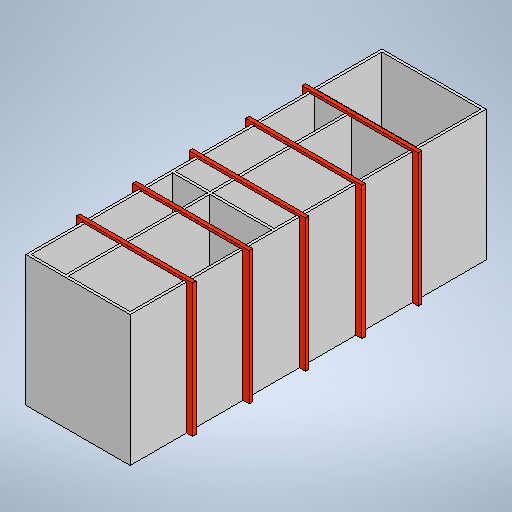
# Autodesk Inventor part: BSH 600 Tank dummy
Saved by Autodesk Inventor 2025.1 (Build 291241020, 241B)
## iProperties
Created: 2024-09-10
Part Number: BSH 600 Tank dummy
Material: Generic
Document SubType Name: Modeling
Designer: admin
Density: 1 g/cm^3
Appearance: Default
Author: admin
Autodesk Inventor part; units mm, degrees
ref_plane "YZ Plane" through (0, 0, 0) normal (1, 0, 0) x (0, 1, 0)
ref_plane "XZ Plane" through (0, 0, 0) normal (0, 1, 0) x (-1, 0, 0)
ref_plane "XY Plane" through (0, 0, 0) normal (0, 0, 1) x (1, 0, 0)
sketch "Sketch1" plane through (0, 0, 0) normal (0, 0, 1) x (1, 0, 0)
  line L0 (1200, 4100) -> (-1200, 4100)
  line L1 (-1200, 4100) -> (-1200, -4100)
  line L2 (-1200, -4100) -> (1200, -4100)
  line L3 (1200, -4100) -> (1200, 4100)
  line L4 (1200, 4100) -> (-1200, -4100) construction
  line L5 (-1200, 4100) -> (1200, -4100) construction
  point P0 (0, 0)
  dimension "d0" = 2400
  dimension "d1" = 8200
  constraints: 12 end point, 2 midpoint, 2 parallel, 1 horizontal, 1 perpendicular
  measures "d0" distance of L2.end L1.end
  measures "d1" distance of L1.end L0.end
extrude "Extrusion1" add sketch "Sketch1" along normal blind 10
sketch "Sketch2" plane through (0, 0, 10) normal (0, 0, 1) x (1, 0, 0)
  line L0 (-1200, 4100) -> (-1200, -4100) projected
  line L1 (-1200, -4100) -> (1200, -4100) projected
  line L2 (1200, -4100) -> (1200, 4100) projected
  line L3 (1200, 4100) -> (-1200, 4100) projected
  line L4 (1140, 4040) -> (1140, -4040)
  line L5 (1140, -4040) -> (-1140, -4040)
  line L6 (-1140, -4040) -> (-1140, 4040)
  line L7 (-1140, 4040) -> (1140, 4040)
  line L8 (1140, 2540) -> (-1140, 2540)
  line L9 (-1140, 2540) -> (-1140, 2480)
  line L10 (-1140, 2480) -> (1140, 2480)
  line L11 (1140, 2480) -> (1140, 2540)
  line L12 (-280, -4040) -> (-340, -4040)
  line L13 (-340, -4040) -> (-340, 2480)
  line L14 (-340, 2480) -> (-280, 2480)
  line L15 (-280, 2480) -> (-280, -4040)
  line L16 (-1140, -720) -> (1140, -720)
  line L17 (1140, -720) -> (1140, -780)
  line L18 (1140, -780) -> (-1140, -780)
  line L19 (-1140, -780) -> (-1140, -720)
  point P0 (0, 0)
  point P1 (-280, -720)
  point P2 (-340, -780)
  point P3 (-1140, -780)
  point P4 (-280, -780)
  point P5 (-340, -720)
  dimension "d4" = 60
  dimension "d5" = 60
  dimension "d6" = 1500
  dimension "d7" = 800
  dimension "d8" = 3200
  constraints: 32 end point, 6 parallel, 5 perpendicular, 4 collinear, 3 horizontal, 2 point on line, 3 other
  measures "d4" distance between parallel lines of L2 L4
  measures "d5" distance between parallel lines of L10 L8
  measures "d6" distance between parallel lines of L8 L7
  measures "d7" distance between parallel lines of L6 L13
  measures "d8" distance between parallel lines of L16 L10
extrude "Extrusion2" add sketch "Sketch2" along normal blind 3000 contours L3 L2 L1 L0 | L4 L10 L6 L8 | L4 L18 L15 L16 | L15 L16 L13 L10 | L15 L18 L13 L16 | L16 L13 L18 L6 | L15 L5 L13 L18
sketch "Sketch5" plane through (-1200, 4100, 0) normal (-1, 0, 0) x (0, 0, 1)
  line L0 (0, 0) -> (0, -8200) projected
  line L1 (0, -8200) -> (3010, -8200) projected
  line L2 (3010, 0) -> (3010, -8200) construction
  line L3 (0, 0) -> (3010, 0) construction
  circle A0 centre (150, -750) radius 38
  circle A1 centre (2660, -1300) radius 45
  circle A2 centre (2390, -6550) radius 38
  circle A3 centre (1400, -750) radius 38
  circle A4 centre (150, -4700) radius 45
  point P0 (0, -4100)
  dimension "d21" = 76
  dimension "d23" = 1300
  dimension "d24" = 350
  dimension "d25" = 90
  dimension "d26" = 150
  dimension "d27" = 1400
  dimension "d28" = 750
  dimension "d29" = 90
  dimension "d30" = 3500
  dimension "d31" = 620
  dimension "d32" = 1650
  constraints: 5 centre point, 2 equal radius, 1 horizontal alignment, 1 vertical alignment
  measures "d21" diameter of A0
  measures "d23" distance from line of L3 A1.centre
  measures "d24" distance from line of A1.centre L2
  measures "d25" diameter of A1
  measures "d26" distance from line of L0 A0.centre
  measures "d27" distance from line of L0 A3.centre
  measures "d28" distance from line of A3.centre L3
  measures "d29" diameter of A4
  measures "d30" distance from line of A4.centre L1
  measures "d31" distance from line of A2.centre L2
  measures "d32" distance from line of L1 A2.centre
sketch "Sketch3" plane through (0, 0, 0) normal (0, 0, 1) x (1, 0, 0)
  line L0 (-1200, 4100) -> (-1200, -4100) construction
  line L1 (1200, 4100) -> (-1200, 4100) construction
  line L2 (1200, -4100) -> (1200, 4100) construction
  line L3 (-1200, -4100) -> (1200, -4100) construction
  line L4 (-1200, 2480) -> (-1340, 2480)
  line L5 (-1340, 2480) -> (-1340, 2400)
  line L6 (-1340, 2400) -> (-1200, 2400)
  line L7 (-1200, 2400) -> (-1200, 2480)
  line L8 (1200, 2480) -> (1340, 2480)
  line L9 (1340, 2480) -> (1340, 2400)
  line L10 (1340, 2400) -> (1200, 2400)
  line L11 (1200, 2400) -> (1200, 2480)
  point P0 (0, 0)
  dimension "d11" = 140
  dimension "d12" = 80
  dimension "d13" = 1620
  constraints: 16 end point, 4 parallel, 2 equal length, 2 horizontal, 2 perpendicular, 2 point on line, 1 collinear
  measures "d11" distance of L6.end L5.end
  measures "d12" distance of L5.end L4.end
  measures "d13" distance between parallel lines of L1 L4
extrude "Extrusion3" add sketch "Sketch3" along normal blind 3000
sketch "Sketch4" plane through (0, 0, 3000) normal (0, 0, 1) x (1, 0, 0)
  line L0 (1200, 2400) -> (1340, 2400) projected
  line L1 (1340, 2400) -> (1340, 2480) projected
  line L2 (1340, 2480) -> (1200, 2480) projected
  line L3 (1200, 2400) -> (1200, 2480) projected
  line L4 (-1340, 2480) -> (-1340, 2400) projected
  line L5 (-1340, 2400) -> (-1200, 2400) projected
  line L6 (-1200, 2480) -> (-1200, 2400) projected
  line L7 (-1200, 2480) -> (-1340, 2480) projected
  line L8 (-1200, 2480) -> (-1340, 2480) projected
  line L9 (1200, 2480) -> (-1200, 2480)
  line L10 (-1200, 2400) -> (1200, 2400)
  line L11 (1200, -4100) -> (1200, 4100) projected
  line L12 (1200, 2480) -> (-1200, 2480)
  point P0 (0, 0)
  constraints: 6 end point, 2 collinear, 1 perpendicular
extrude "Extrusion4" add sketch "Sketch4" along normal blind 60
pattern_linear "Rectangular Pattern1" count 5 spacing 1300 along (0, -1, 0) of "Extrusion3", "Extrusion4"
extrude "Extrusion5" add sketch "Sketch5" along normal blind 100
equation "\"d5\" = d4"
body "Solid1"
